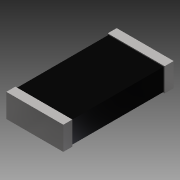
# Autodesk Inventor part: s174 Resistor
Saved by Autodesk Inventor 2015 (Build 190159000, 159)
## iProperties
Created: 2016-01-19
Part Number: s174 Resistor
Material: Generic
Document SubType Name: Modeling
Designer: Kyle
Density: 1 g/cm^3
Appearance: Default
Author: Kyle
Autodesk Inventor part; units mm, degrees
ref_plane "YZ Plane" through (0, 0, 0) normal (1, 0, 0) x (0, 1, 0)
ref_plane "XZ Plane" through (0, 0, 0) normal (0, 1, 0) x (-1, 0, 0)
ref_plane "XY Plane" through (0, 0, 0) normal (0, 0, 1) x (1, 0, 0)
sketch "Sketch1" plane through (0, 0, 0) normal (0, 0, 1) x (1, 0, 0)
  line L0 (0, 0) -> (1.5494, 0)
  line L1 (1.5494, 0) -> (1.5494, 0.6096)
  line L2 (1.5494, 0.6096) -> (0, 0.6096)
  line L3 (0, 0.6096) -> (0, 0)
  dimension "d0" = 0.6096
  dimension "d1" = 1.5494
  constraints: 8 end point, 2 parallel, 1 horizontal, 1 perpendicular
  measures "d0" distance of L0.end L1.end
  measures "d1" distance of L1.end L2.end
extrude "Extrusion1" add sketch "Sketch1" along normal blind 2.5908
sketch "Sketch2" plane through (0, 0, 2.5908) normal (0, 0, 1) x (1, 0, 0)
  line L0 (-0.0254, 0.635) -> (1.5748, 0.635)
  line L1 (1.5748, 0.635) -> (1.5748, -0.0254)
  line L2 (1.5748, -0.0254) -> (-0.0254, -0.0254)
  line L3 (-0.0254, -0.0254) -> (-0.0254, 0.635)
  line L4 (1.5494, 0) -> (1.5494, 0.6096) projected
  line L5 (0, 0.6096) -> (0, 0) projected
  line L6 (1.5494, 0.6096) -> (0, 0.6096) projected
  line L7 (0, 0) -> (1.5494, 0) projected
  dimension "d4" = 0.0254
  dimension "d5" = 0.0254
  dimension "d6" = 0.0254
  dimension "d7" = 0.0254
  constraints: 8 end point, 2 parallel, 1 horizontal, 1 perpendicular
  measures "d4" distance between parallel lines of L1 L4
  measures "d5" distance between parallel lines of L3 L5
  measures "d6" distance between parallel lines of L0 L6
  measures "d7" distance between parallel lines of L2 L7
extrude "Extrusion2" add sketch "Sketch2" along normal blind 0.254 contours L0 L1 L2 L3 | L7 L5 L6 L4
sketch "Sketch3" plane through (0, 0, 0) normal (0, 0, -1) x (-1, 0, 0)
  line L0 (0.0254, -0.0254) -> (-1.5748, -0.0254)
  line L1 (-1.5748, -0.0254) -> (-1.5748, 0.635)
  line L2 (-1.5748, 0.635) -> (0.0254, 0.635)
  line L3 (0.0254, 0.635) -> (0.0254, -0.0254)
  point P0 (0, 0)
  constraints: 8 end point, 2 parallel, 1 horizontal, 1 perpendicular
extrude "Extrusion3" add sketch "Sketch3" along normal blind 0.254
body "Solid1"
